Autodesk Inventor part; units mm, degrees
(part 2 of 2)
sketch "Sketch18" plane through (0, 5, 0) normal (0, -1, 0) x (1, 0, 0)
  circle A0 centre (0, 0) radius 4
  dimension "d63" = 8
  constraints: 1 centre point, 1 coincident
  measures "d63" diameter of A0
extrude "Extrusion10" cut sketch "Sketch18" against normal up to next
body "Solid1"
